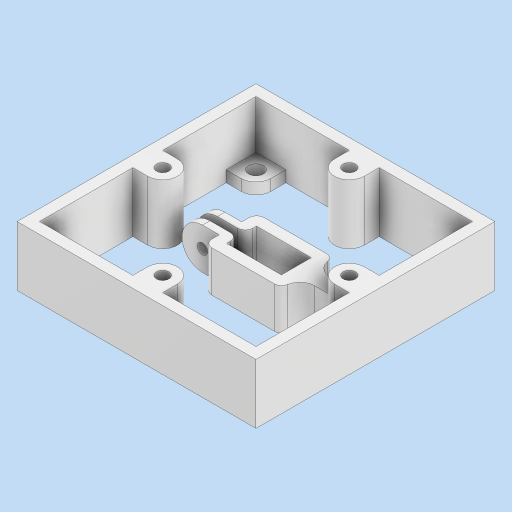
# Autodesk Inventor part: Frame_FS90R
Saved by Autodesk Inventor 2024 (Build 280153000, 153)
## iProperties
Created: 2023-04-24
Part Number: Frame_FS90R
Material: ABS Plastic
Document SubType Name: Modeling
Designer: byrne
Density: 1.06 g/cm^3
Appearance: Smooth - White
Author: byrne
Autodesk Inventor part; units mm, degrees
note: some values were not read from the file. Chosen so that the rebuilt part matches the saved one: direction of "Hole4".
ref_plane "YZ Plane" through (0, 0, 0) normal (1, 0, 0) x (0, 1, 0)
ref_plane "XZ Plane" through (0, 0, 0) normal (0, 1, 0) x (-1, 0, 0)
ref_plane "XY Plane" through (0, 0, 0) normal (0, 0, 1) x (1, 0, 0)
sketch "Sketch3" plane through (0, 0, 0) normal (0, 1, 0) x (-1, 0, 0)
  line L0 (-50.8, 50.8) -> (50.8, 50.8)
  line L1 (50.8, 50.8) -> (50.8, -50.8)
  line L2 (50.8, -50.8) -> (-50.8, -50.8)
  line L3 (-50.8, -50.8) -> (-50.8, 50.8)
  line L4 (-50.8, 50.8) -> (50.8, -50.8) construction
  line L5 (50.8, 50.8) -> (-50.8, -50.8) construction
  line L6 (-46.0375, 46.0375) -> (46.0375, 46.0375)
  line L7 (46.0375, 46.0375) -> (46.0375, -46.0375)
  line L8 (46.0375, -46.0375) -> (-46.0375, -46.0375)
  line L9 (-46.0375, -46.0375) -> (-46.0375, 46.0375)
  point P0 (0, 0)
  dimension "d17" = 101.6
  dimension "d18" = 101.6
  dimension "d19" = 4.7625
  constraints: 20 end point, 4 parallel, 2 midpoint, 2 perpendicular, 1 horizontal, 3 other
  measures "d17" distance of L1.end L2.end
  measures "d18" distance of L0.end L1.end
  measures "d19" distance between parallel lines of L3 L9
extrude "Exterior Wall" add sketch "Sketch3" along normal blind 25.4
sketch "Sketch4" plane through (0, 0, 0) normal (0, -1, 0) x (1, 0, 0)
  line L0 (-50.8, 50.8) -> (50.8, 50.8)
  line L1 (50.8, 50.8) -> (50.8, -50.8)
  line L2 (50.8, -50.8) -> (-50.8, -50.8)
  line L3 (-50.8, -50.8) -> (-50.8, 50.8)
  line L4 (-50.8, 50.8) -> (50.8, -50.8) construction
  line L5 (50.8, 50.8) -> (-50.8, -50.8) construction
  line L6 (46.0375, -46.0375) -> (46.0375, 46.0375)
  line L7 (46.0375, 46.0375) -> (-46.0375, 46.0375)
  line L8 (-46.0375, 46.0375) -> (-46.0375, -46.0375)
  line L9 (-46.0375, -46.0375) -> (46.0375, -46.0375)
  circle A0 centre (39.6875, 39.6875) radius 3.175
  circle A1 centre (39.6875, 39.6875) radius 6.35
  line L10 (33.3375, 33.3375) -> (33.3159, 33.3375)
  line L11 (33.3375, 39.6875) -> (33.3375, 46.0375)
  line L12 (46.0375, 33.3375) -> (39.6875, 33.3375)
  point P0 (0, 0)
  dimension "d22" = 101.6
  dimension "d23" = 101.6
  dimension "d24" = 4.7625
  dimension "d25" = 6.35
  dimension "d26" = 3.175
  constraints: 26 end point, 5 tangent, 4 parallel, 3 horizontal, 3 point on line, 2 centre point, 2 midpoint, 2 perpendicular, 2 point on circle, 1 vertical, 3 other
  measures "d22" distance of L1.end L2.end
  measures "d23" distance of L0.end L1.end
  measures "d24" distance between parallel lines of L1 L6
  measures "d25" diameter of A0
  measures "d26" radial gap between concentric circles of A0 A1
extrude "Mounting Hole" add sketch "Sketch4" against normal blind 4.7625 contours L12 A1 L6 | A1 L7 L6 | A1 | A1 L11 L7
pattern_circular "Mounting Hole Pattern" count 4 over 360 about axis through (0, -10, 0) along (0, 1, 0) of "Mounting Hole"
sketch "Sketch17" plane through (0, 0, 0) normal (0, -1, 0) x (1, 0, 0)
  line L0 (16.95, -6.15) -> (-5.9, -6.15) construction
  line L1 (-5.9, -6.15) -> (-5.9, 6.15) construction
  line L2 (-5.9, 6.15) -> (16.95, 6.15) construction
  line L3 (16.95, 6.15) -> (16.95, -6.15) construction
  line L4 (-6.1, -6.35) -> (17.15, -6.35)
  line L5 (17.15, -6.35) -> (17.15, 6.35)
  line L6 (17.15, 6.35) -> (-6.1, 6.35)
  line L7 (-6.1, 6.35) -> (-6.1, -6.35)
  circle A0 centre (-39.6875, 39.6875) radius 3.175 projected
  circle A1 centre (-39.6875, -39.6875) radius 3.175 projected
  circle A2 centre (39.6875, -39.6875) radius 3.175 projected
  circle A3 centre (39.6875, 39.6875) radius 3.175 projected
  line L8 (50.8, -50.8) -> (-50.8, -50.8) projected
  line L9 (50.8, 50.8) -> (50.8, -50.8) projected
  line L10 (-50.8, 50.8) -> (50.8, 50.8) projected
  line L11 (-50.8, -50.8) -> (-50.8, 50.8) projected
  line L12 (-33.3375, -46.0375) -> (33.3375, -46.0375) projected
  line L13 (-33.3375, -46.0375) -> (-33.3375, -39.6875) projected
  arc A4 (-33.3375, -39.6875) -> (-39.6875, -33.3375) centre (-39.6875, -39.6875) ccw projected
  line L14 (-39.6875, -33.3375) -> (-46.0375, -33.3375) projected
  line L15 (-46.0375, 33.3375) -> (-46.0375, -33.3375) projected
  line L16 (-46.0375, 33.3375) -> (-39.6875, 33.3375) projected
  arc A5 (-39.6875, 33.3375) -> (-33.3375, 39.6875) centre (-39.6875, 39.6875) ccw projected
  line L17 (-33.3375, 39.6875) -> (-33.3375, 46.0375) projected
  line L18 (33.3375, 46.0375) -> (-33.3375, 46.0375) projected
  line L19 (33.3375, 46.0375) -> (33.3375, 39.6875) projected
  arc A6 (33.3375, 39.6875) -> (39.6875, 33.3375) centre (39.6875, 39.6875) ccw projected
  line L20 (39.6875, 33.3375) -> (46.0375, 33.3375) projected
  line L21 (46.0375, -33.3375) -> (46.0375, 33.3375) projected
  line L22 (46.0375, -33.3375) -> (39.6875, -33.3375) projected
  arc A7 (39.6875, -33.3375) -> (33.3375, -39.6875) centre (39.6875, -39.6875) ccw projected
  line L23 (33.3375, -39.6875) -> (33.3375, -46.0375) projected
  line L24 (21.9125, -11.1125) -> (-10.8625, -11.1125)
  line L25 (-10.8625, -11.1125) -> (-10.8625, 11.1125)
  line L26 (-10.8625, 11.1125) -> (21.9125, 11.1125)
  line L27 (21.9125, 11.1125) -> (21.9125, -11.1125)
  line L28 (46.0375, -3.175) -> (21.9125, -3.175)
  line L29 (21.9125, -3.175) -> (21.9125, 3.175)
  line L30 (21.9125, 3.175) -> (46.0375, 3.175)
  line L31 (46.0375, 3.175) -> (46.0375, -3.175)
  line L32 (-26.7375, 4.7625) -> (-6.1, 4.7625)
  line L33 (-6.1, 4.7625) -> (-6.1, 1.5875)
  line L34 (-6.1, 1.5875) -> (-26.7375, 1.5875)
  line L35 (-26.7375, 1.5875) -> (-26.7375, 4.7625)
  line L36 (-26.7375, -1.5875) -> (-6.1, -1.5875)
  line L37 (-6.1, -1.5875) -> (-6.1, -4.7625)
  line L38 (-6.1, -4.7625) -> (-26.7375, -4.7625)
  line L39 (-26.7375, -4.7625) -> (-26.7375, -1.5875)
  line L40 (-16.4188, 1.5875) -> (-16.4188, -1.5875) construction
  point P0 (0, 0)
  point P1 (-5.9, 0)
  point P2 (21.9125, 0)
  point P3 (46.0375, 0)
  point P4 (-16.4188, 0)
  point P5 (-10.8625, 0)
  point P6 (-10.8625, -4.7625)
  point P7 (-10.8625, -1.5875)
  point P8 (-10.8625, 1.5875)
  point P9 (-10.8625, 4.7625)
  point P10 (-6.1, 1.5875)
  dimension "d139" = 5.9
  dimension "d140" = 12.3
  dimension "d141" = 22.85
  dimension "d142" = 0.2
  dimension "d143" = 4.7625
  dimension "d144" = 6.35
  dimension "d165" = 3.175
  dimension "d166" = 3.175
  dimension "d167" = 20.6375
  constraints: 50 end point, 12 parallel, 9 midpoint, 6 perpendicular, 4 horizontal, 2 collinear, 2 equal length, 2 horizontal alignment, 6 other
  measures "d139" distance from line of L1 point (0, 0)
  measures "d140" distance between parallel lines of L0 L2
  measures "d141" distance between parallel lines of L1 L3
  measures "d142" distance between parallel lines of L0 L4
  measures "d143" distance between parallel lines of L4 L24
  measures "d144" distance between parallel lines of L30 L28
  measures "d165" distance between parallel lines of L36 L34
  measures "d166" distance between parallel lines of L34 L32
  measures "d167" distance of L32.start L32.end
extrude "Servo Mount" add sketch "Sketch17" against normal blind 17.4625 contours L4 L5 L6 L7 L32 L25 L26 L27 L24 L38 | L38 L25 L36 L7 | L38 L39 L36 L25 | L34 L25 L32 L7 | L34 L35 L32 L25 | L27 L30 L21 L28
fillet "Servo Mount Fillet 1" radius 6.35 2 edges at (21.9125, 8.7313, -3.175) (21.9125, 8.7313, 3.175)
fillet "Servo Mount Fillet 2" radius 3.175 6 edges at (21.9125, 8.7313, -11.1125) (-10.8625, 8.7313, -11.1125) (-10.8625, 8.7313, 11.1125) (21.9125, 8.7313, 11.1125) (-6.1, 8.7313, -1.5875) (-6.1, 8.7313, 1.5875)
sketch "Sketch18" plane through (0, 25.4, 0) normal (0, 1, 0) x (1, 0, 0)
  line L0 (50.8, 50.8) -> (-50.8, 50.8) projected
  line L1 (-50.8, 50.8) -> (-50.8, -50.8) projected
  line L2 (-50.8, -50.8) -> (50.8, -50.8) projected
  line L3 (50.8, -50.8) -> (50.8, 50.8) projected
  line L4 (46.0375, -46.0375) -> (-46.0375, -46.0375) projected
  line L5 (-46.0375, -46.0375) -> (-46.0375, 46.0375) projected
  line L6 (-46.0375, 46.0375) -> (46.0375, 46.0375) projected
  line L7 (46.0375, 46.0375) -> (46.0375, -46.0375) projected
  circle A0 centre (-39.6875, 0) radius 6.35
  line L8 (-46.0375, -6.35) -> (-39.6875, -6.35)
  line L9 (-39.6875, 6.35) -> (-46.0375, 6.35)
  point P0 (0, 0)
  point P1 (-46.0375, 0)
  dimension "d152" = 12.7
  constraints: 4 end point, 3 tangent, 2 horizontal, 2 point on circle, 2 point on line, 1 centre point, 1 coincident, 1 horizontal alignment, 1 midpoint
  measures "d152" diameter of A0
extrude "Cover Mounting Block" add sketch "Sketch18" against normal blind 25.4 contours L5 A0 L8 | L5 L9 A0 | A0
hole "Cover Mounting Hole" at (-39.6875, 25.4, 0) direction (0, -1, 0) diameter 5.334 end through all
pattern_circular "Cover Mounting Pattern" count 4 over 360 about axis through (0, -10, 0) along (0, 1, 0) of "Cover Mounting Block", "Cover Mounting Hole"
fillet "Fillet15" radius 8.7313 4 edges at (-26.7375, 17.4625, 3.175) (-26.7375, 0, 3.175) (-26.7375, 0, -3.175) (-26.7375, 17.4625, -3.175)
sketch "Sketch19" plane through (-10.8625, 0, 4.7625) normal (0, 0, 1) x (1, 0, 0)
  arc A0 (-7.1438, 17.4625) -> (-7.1438, 0) centre (-7.1438, 8.7313) ccw projected
  point P0 (10.8625, 0)
  constraints: 1 coincident
hole "Hole4" at (-18.0063, 8.7313, 4.7625) direction (0, 0, -1) diameter 4.445 depth 9.525
body "Solid2"
